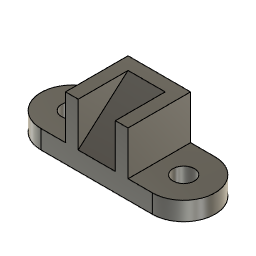
A2 (Autodesk Fusion 360 design; units mm, degrees)
Autodesk Fusion 360 part; units mm, degrees
note: some values were not read from the file. Chosen so that the rebuilt part matches the saved one: which pieces of a blend or face edit are solid.
sketch "Sketch1" plane through (0, 0, 0) normal (0, 0, 1) x (1, 0, 0)
  line L0 (-50, 25) -> (64, 25)
  line L1 (64, 25) -> (64, -39)
  line L2 (64, -39) -> (-50, -39)
  line L3 (-50, -39) -> (-50, 25)
  arc A0 (64, -39) -> (64, 25) centre (64, -7) ccw
  arc A1 (-50, 25) -> (-50, -39) centre (-50, -7) ccw
  line L4 (-50, -39) -> (26, -39)
  line L5 (64, -39) -> (-12, -39)
  line L6 (26, -39) -> (-12, -39)
  line L7 (-12, -39) -> (-12, 25)
  line L8 (-12, 25) -> (26, 25)
  line L9 (26, 25) -> (26, -39)
  line L10 (-50, 25) -> (39, 25)
  line L11 (64, 25) -> (-25, 25)
  line L12 (-25, 25) -> (39, 25)
  line L13 (39, 25) -> (39, -39)
  line L14 (39, -39) -> (-25, -39)
  line L15 (-25, -39) -> (-25, 25)
  circle A2 centre (64, -7) radius 11
  circle A3 centre (-50, -7) radius 11
  dimension "d1" = 114
  dimension "d2" = 64
  dimension "d3" = 76
  dimension "d4" = 76
  dimension "d5" = 89
  dimension "d6" = 89
  dimension "d7" = 64
  dimension "d8" = 22
  dimension "d9" = 22
  constraint horizontal L0
  constraint vertical L1
  constraint horizontal L2
  constraint vertical L3
  constraint tangent L0 A0
  constraint tangent L0 A1
  constraint perpendicular L3 L4
  constraint midpoint L4 L5.end
  constraint horizontal L6
  constraint vertical L7
  constraint horizontal L8
  constraint vertical L9
  constraint coincident L0 L7.end
  constraint perpendicular L9 L10
  constraint perpendicular L1 L11
  constraint horizontal L12
  constraint vertical L13
  constraint horizontal L14
  constraint vertical L15
  constraint concentric A0 A2
  constraint concentric A1 A3
  measures "d1" distance of L0.start L0.end
  measures "d2" distance of L0.start L2.end
  measures "d3" distance of L2.end L4.end
  measures "d4" distance of L1.end L5.end
  measures "d5" distance of L0.start L10.end
  measures "d6" distance of L0.end L11.end
  measures "d7" distance of L11.end L10.end
  measures "d8" diameter of A2
  measures "d9" diameter of A3
extrude "Extrude4" add sketch "Sketch1" along normal blind 64 contours L0 L2 L4 L7 L10 L11 L12 L14 L15 | L0 L2 L5 L9 L10 L11 L12 L13 L14 makes body 1 at (-12, -17.6667, 21.3333) makes body 2 at (39, 3.6667, 21.3333)
extrude "Extrude5" add sketch "Sketch1" along normal blind 19 separate body contours L0 L2 L3 L4 L10 L15 A3 | L3 A1 A3 | L0 L1 L2 L5 L11 L13 A2 | L1 A0 A2 makes body 3 at (53.8333, -31.5088, 0) makes body 4 at (-39.8333, 17.5088, 0)
sketch "Sketch2" plane through (0, 0, 0) normal (0, 0, 1) x (1, 0, 0)
  line L0 (-12, 25) -> (26, 25)
  line L1 (26, 25) -> (26, 12)
  line L2 (26, 12) -> (-12, 12)
  line L3 (-12, 12) -> (-12, 25)
  line L4 (-12, 12) -> (26, 12)
  line L5 (26, 12) -> (26, -39)
  line L6 (26, -39) -> (-12, -39)
  line L7 (-12, -39) -> (-12, 12)
  dimension "d22" = 13
  dimension "d23" = 51
  constraint horizontal L0
  constraint vertical L1
  constraint horizontal L2
  constraint vertical L3
  constraint horizontal L4
  constraint vertical L5
  constraint horizontal L6
  constraint vertical L7
  measures "d22" distance of L0.start L2.end
  measures "d23" distance of L2.end L6.end
extrude "Extrude6" add sketch "Sketch2" along normal blind 64 separate body contours L0 L1 L2 L3 L4 makes body 5
extrude "Extrude8" cut 1 faces at (0.6667, 20.6667, 0) along direction (0, 0, -1) blind -19 and the other way blind 0 on bodies 5 bodies 5
extrude "Extrude9" add sketch "Sketch1" along normal blind 19 contours L0 L2 L4 L5 L6 L7 L8 L9 L10 L11 L12 L14 bodies 5
draft "Draft1" angle 48.576 neutral plane through (0, 0, 64) pull (0, 0, 1) 1 faces at (13.3333, 12, 34) on bodies 5
combine "Combine1" operation add target body 4 tool bodies 3 5 1 2
named bodies: "A2"
